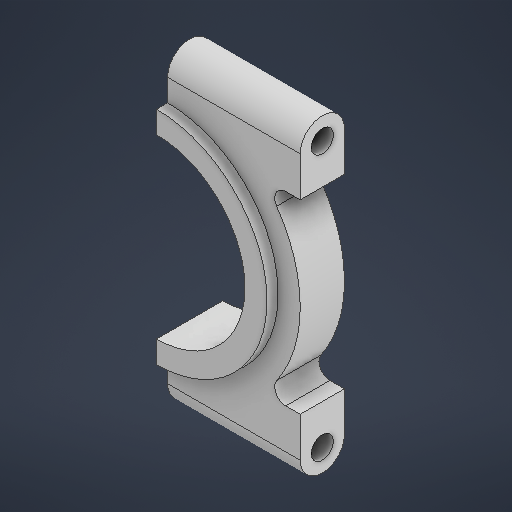
# Autodesk Inventor part: rodcap
Saved by Autodesk Inventor 2026.1 (Build 301233020, 233B)
## iProperties
Created: 2025-11-21
Part Number: rodcap
Material: Generic
Document SubType Name: Modeling
Designer: ender
Density: 1 g/cm^3
Appearance: Default
Author: ender
Autodesk Inventor part; units mm, degrees
ref_plane "YZ Plane" through (0, 0, 0) normal (1, 0, 0) x (0, 1, 0)
ref_plane "XZ Plane" through (0, 0, 0) normal (0, 1, 0) x (-1, 0, 0)
ref_plane "XY Plane" through (0, 0, 0) normal (0, 0, 1) x (1, 0, 0)
sketch "Sketch1" plane through (0, 0, 0) normal (0, 0, 1) x (1, 0, 0)
  arc A0 (0, -25.4) -> (0, 25.4) centre (0, 0) ccw
  line L0 (0, 25.4) -> (0, 44.45)
  line L1 (0, 44.45) -> (38.1, 44.45)
  line L2 (38.1, 44.45) -> (38.1, -44.45)
  line L3 (38.1, -44.45) -> (0, -44.45)
  line L4 (0, -44.45) -> (0, -25.4)
  dimension "d1" = 44.45
  dimension "d2" = 38.1
  dimension "d3" = 88.9
  dimension "d4" = 25.4
  constraints: 10 end point, 3 perpendicular, 2 point on circle, 1 centre point, 1 coincident, 1 collinear, 1 horizontal, 1 point on line, 1 vertical
  measures "d1" distance of A0.centre L0.end
  measures "d2" distance of L0.end L1.end
  measures "d3" distance of L1.end L2.end
  measures "d4" radius of A0
extrude "Extrusion1" add sketch "Sketch1" along normal mid plane 12.7
sketch "Sketch2" plane through (0, 0, 6.35) normal (0, 0, 1) x (1, 0, 0)
  line L0 (38.1, -44.45) -> (38.1, 44.45) projected
  line L1 (38.1, 26.67) -> (27.2088, 26.67)
  line L2 (38.1, 44.45) -> (0, 44.45) projected
  line L3 (38.1, -26.67) -> (27.2088, -26.67)
  line L4 (0, -44.45) -> (38.1, -44.45) projected
  arc A0 (27.2088, -26.67) -> (27.2088, 26.67) centre (0, 0) ccw
  point P0 (38.1, 0)
  dimension "d7" = 17.78
  dimension "d9" = 38.1
  constraints: 4 end point, 2 point on circle, 2 point on line, 1 centre point, 1 coincident, 1 horizontal, 1 parallel, 1 perpendicular
  measures "d7" distance between parallel lines of L2 L1
  measures "d9" radius of A0
extrude "Extrusion2" cut sketch "Sketch2" against normal through all
sketch "Sketch3" plane through (0, 0, 0) normal (0, 0, 1) x (1, 0, 0)
  arc A0 (0, -31.75) -> (0, 31.75) centre (0, 0) ccw
  arc A1 (0, -25.4) -> (0, 25.4) centre (0, 0) ccw projected
  line L0 (0, 25.4) -> (0, 31.75)
  line L1 (0, 25.4) -> (0, 44.45) projected
  line L2 (0, -25.4) -> (0, -31.75)
  line L3 (0, -44.45) -> (0, -25.4) projected
  line L4 (0, 25.4) -> (0, 31.75)
  line L5 (0, -31.75) -> (0, -25.4)
  dimension "d14" = 31.75
  constraints: 8 end point, 2 collinear, 2 point on circle, 2 point on line, 1 centre point, 1 coincident
  measures "d14" radius of A0
extrude "Extrusion3" add sketch "Sketch3" along normal mid plane 19.05
fillet "Fillet1" radius 3.175 2 edges at (27.2088, -26.67, 0) (27.2088, 26.67, 0)
fillet "Fillet2" radius 6.35 4 edges at (19.05, 44.45, 6.35) (19.05, 44.45, -6.35) (19.05, -44.45, 6.35) (19.05, -44.45, -6.35)
sketch "Sketch4" plane through (38.1, -26.67, 6.35) normal (1, 0, 0) x (0, 0, -1)
  circle A0 centre (6.35, 64.77) radius 3.175
  circle A1 centre (6.35, -11.43) radius 3.175
  arc A2 (0, -11.43) -> (12.7, -11.43) centre (6.35, -11.43) ccw projected
  arc A3 (12.7, 64.77) -> (0, 64.77) centre (6.35, 64.77) ccw projected
  point P0 (6.35, 26.67)
  dimension "d19" = 6.35
  constraints: 2 centre point, 2 concentric, 1 equal radius
  measures "d19" diameter of A0
extrude "Extrusion4" cut sketch "Sketch4" against normal through all
body "Solid1"
